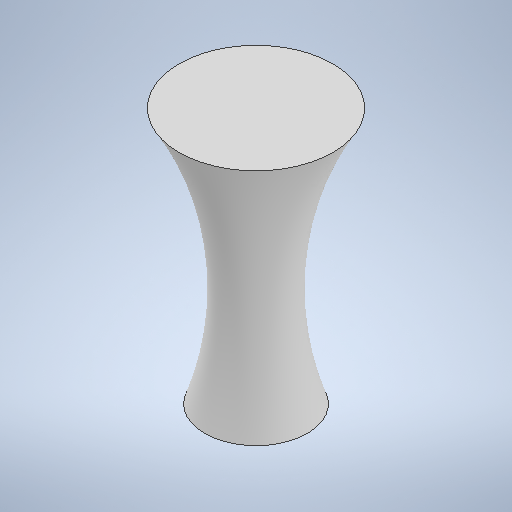
# Autodesk Inventor part: 4xDisplay
Saved by Autodesk Inventor 2025.3 (Build 293356000, 356)
## iProperties
Created: 2025-06-26
Part Number: 4xDisplay
Material: Generic
Document SubType Name: Modeling
Designer: user
Density: 1 g/cm^3
Appearance: Default
Author: user
Autodesk Inventor part; units mm, degrees
ref_plane "YZ Plane" through (0, 0, 0) normal (1, 0, 0) x (0, 1, 0)
ref_plane "XZ Plane" through (0, 0, 0) normal (0, 1, 0) x (-1, 0, 0)
ref_plane "XY Plane" through (0, 0, 0) normal (0, 0, 1) x (1, 0, 0)
sketch "Sketch1" plane through (0, 0, 0) normal (1, 0, 0) x (0, 1, 0)
  line L0 (0, 200) -> (0, -200)
  line L1 (0, 0) -> (1000, 0)
  line L2 (1000, 300) -> (1000, -300)
  arc A0 (0, 200) -> (1000, 300) centre (391.5683, 1334.3166) ccw
  dimension "d0" = 400
  dimension "d1" = 1000
  dimension "d2" = 600
  dimension "d3" = 1200
  constraints: 6 end point, 2 midpoint, 2 point on circle, 2 vertical, 1 centre point, 1 coincident, 1 horizontal
  measures "d0" distance of L0.start L0.end
  measures "d1" distance of L1.end L1.start
  measures "d2" distance of L2.start L2.end
  measures "d3" radius of A0
revolve "Revolution1" add sketch "Sketch1" angle 360 about axis through (0, 0, 0) along (0, 1, 0)
body "Solid1"
